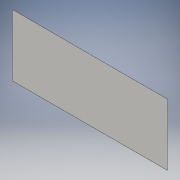
# Autodesk Inventor part: vrRig_v01r1_screenFlat
Saved by Autodesk Inventor 2016 (Build 200138000, 138)
## iProperties
Created: 2019-01-07
Part Number: vrRig_v01r1_screenFlat
Material: Generic
Document SubType Name: Modeling
Designer: harveylab
Density: 1 g/cm^3
Appearance: Default
Author: harveylab
Autodesk Inventor part; units mm, degrees
ref_plane "YZ Plane" through (0, 0, 0) normal (1, 0, 0) x (0, 1, 0)
ref_plane "XZ Plane" through (0, 0, 0) normal (0, 1, 0) x (-1, 0, 0)
ref_plane "XY Plane" through (0, 0, 0) normal (0, 0, 1) x (1, 0, 0)
sketch "Sketch1" plane through (0, 0, 0) normal (0, 0, 1) x (1, 0, 0)
  line L0 (-15.6362, 11.4255) -> (525.3838, 11.4255)
  line L1 (525.3838, 11.4255) -> (525.3838, -204.4745)
  line L2 (525.3838, -204.4745) -> (-15.6362, -204.4745)
  line L3 (-15.6362, -204.4745) -> (-15.6362, 11.4255)
  point P0 (0, 0)
  dimension "d0" = 541.02
  dimension "d1" = 215.9
  constraints: 8 end point, 2 parallel, 1 horizontal, 1 perpendicular
  measures "d0" distance of L1.end L2.end
  measures "d1" distance of L0.end L1.end
extrude "Extrusion1" add sketch "Sketch1" along normal blind 0.254
body "Solid1"
